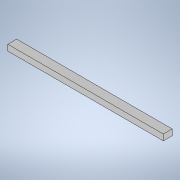
# Autodesk Inventor part: VerstaerkungUnten
Saved by Autodesk Inventor 2020.3 (Build 243373010, 373A)
## iProperties
Created: 2021-02-15
Part Number: VerstaerkungUnten
Material: Generisch
Document SubType Name: Modeling
Designer: Stefan
Density: 1 g/cm^3
Appearance: Vorgabe
Author: Stefan
Autodesk Inventor part; units mm, degrees
ref_plane "YZ Plane" through (0, 0, 0) normal (1, 0, 0) x (0, 1, 0)
ref_plane "XZ Plane" through (0, 0, 0) normal (0, 1, 0) x (-1, 0, 0)
ref_plane "XY Plane" through (0, 0, 0) normal (0, 0, 1) x (1, 0, 0)
sketch "Skizze1" plane through (0, 0, 0) normal (0, 1, 0) x (-1, 0, 0)
  line L0 (38.2353, 18.9706) -> (-487.7647, 18.9706)
  line L1 (-487.7647, 18.9706) -> (-487.7647, -11.0294)
  line L2 (-487.7647, -11.0294) -> (38.2353, -11.0294)
  line L3 (38.2353, -11.0294) -> (38.2353, 18.9706)
  point P0 (0, 0)
  dimension "d0" = 30
  dimension "d1" = 526
  constraints: 8 end point, 2 parallel, 1 horizontal, 1 perpendicular
  measures "d0" distance of L2.end L0.start
  measures "d1" distance of L0.start L0.end
extrude "Extrusion1" add sketch "Skizze1" along normal blind 20
